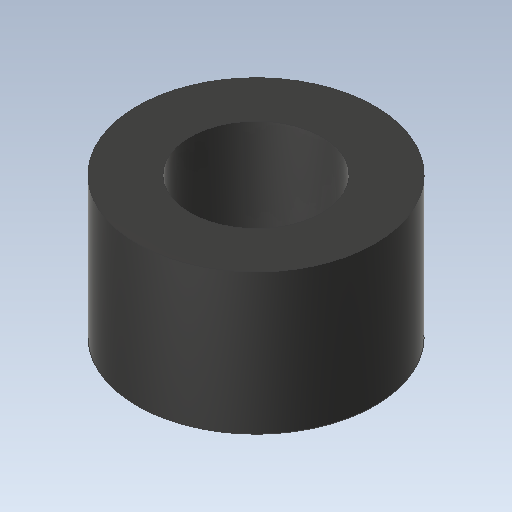
# Autodesk Inventor part: 付け根_サブフレーム_6_4
Saved by Autodesk Inventor 2020 (Build 240168000, 168)
## iProperties
Created: 2016-08-23
Part Number: 付け根_サブフレーム_6_4
Material: アセタール樹脂、黒
Document SubType Name: Modeling
Designer: hiro
Density: 1.425 g/cm^3
Appearance: 滑らか - 黒
Mass: 0.609551 g
Surface Area: 4.80805 cm^2
Volume: 0.427755 cm^3
Category: 付け根
Author: hiro
Autodesk Inventor part; units mm, degrees
ref_plane "YZ Plane" through (0, 0, 0) normal (1, 0, 0) x (0, 1, 0)
ref_plane "XZ Plane" through (0, 0, 0) normal (0, 1, 0) x (-1, 0, 0)
ref_plane "XY Plane" through (0, 0, 0) normal (0, 0, 1) x (1, 0, 0)
sketch "スケッチ1" plane through (0, 0, 0) normal (0, 0, 1) x (1, 0, 0)
  line L0 (3.05, 3.25) -> (5.5, 3.25)
  line L1 (5.5, 3.25) -> (5.5, -3.25)
  line L2 (5.5, -3.25) -> (3.05, -3.25)
  line L3 (3.05, -3.25) -> (3.05, 3.25)
  line L4 (0, 12.2609) -> (0, -12.2609) construction
  point P0 (0, 0)
  point P1 (3.05, 0)
  point P2 (0, 0)
  dimension "d0" = 6.1
  dimension "d1" = 11
  dimension "d2" = 6.5
  constraints: 10 end point, 2 midpoint, 2 parallel, 1 coincident, 1 horizontal, 1 horizontal alignment, 1 perpendicular, 1 vertical
  measures "d0" diameter of L3 L4
  measures "d1" diameter of L1 L4
  measures "d2" distance of L0.end L1.end
revolve "回転1" add sketch "スケッチ1" angle 360 about axis through (0, 12.2609, 0) along (0, -1, 0)
